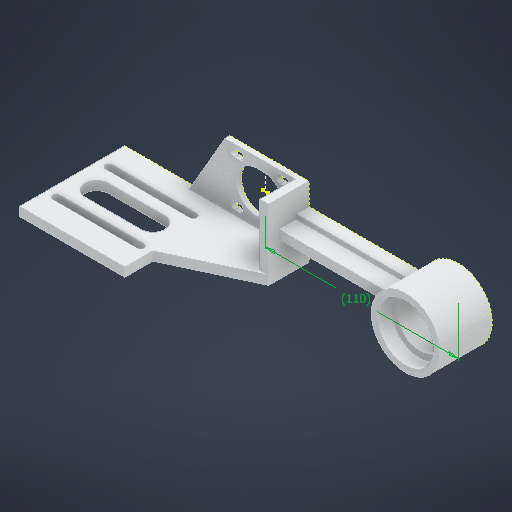
# Autodesk Inventor part: SupportV2_P2
Saved by Autodesk Inventor 2026.2 (Build 302298000, 298)
## iProperties
Created: 2023-04-27
Part Number: SupportV2_P2
Material: PET Plastic
Document SubType Name: Modeling
Designer: Vinicius Silva
Density: 1.541 g/cm^3
Appearance: White
Author: Vinicius Silva
Autodesk Inventor part; units mm, degrees
ref_plane "YZ Plane" through (0, 0, 0) normal (1, 0, 0) x (0, 1, 0)
ref_plane "XZ Plane" through (0, 0, 0) normal (0, 1, 0) x (-1, 0, 0)
ref_plane "XY Plane" through (0, 0, 0) normal (0, 0, 1) x (1, 0, 0)
sketch "Sketch1" plane through (0, 0, 0) normal (0, 0, 1) x (1, 0, 0)
  line L0 (0, 0) -> (30, 0)
  line L1 (30, 0) -> (30, 60)
  line L2 (30, 60) -> (0, 60)
  line L3 (6, 45) -> (24, 45) construction
  line L4 (6, 43) -> (24, 43)
  line L5 (24, 47) -> (6, 47)
  arc A0 (24, 43) -> (24, 47) centre (24, 45) ccw
  line L6 (6, 15) -> (24, 15) construction
  line L7 (6, 13) -> (24, 13)
  line L8 (24, 17) -> (6, 17)
  arc A1 (24, 13) -> (24, 17) centre (24, 15) ccw
  line L9 (0, 30) -> (16, 30) construction
  arc A2 (16, 23.25) -> (16, 36.75) centre (16, 30) ccw
  line L10 (0, 0) -> (-30, 0)
  line L11 (-30, 0) -> (-30, 60)
  line L12 (-30, 60) -> (0, 60)
  line L13 (-6, 45) -> (-24, 45) construction
  line L14 (24, 43) -> (-24, 43)
  line L15 (-24, 47) -> (24, 47)
  arc A3 (-24, 47) -> (-24, 43) centre (-24, 45) ccw
  line L16 (-6, 15) -> (-24, 15) construction
  line L17 (24, 13) -> (-24, 13)
  line L18 (-24, 17) -> (24, 17)
  arc A4 (-24, 17) -> (-24, 13) centre (-24, 15) ccw
  line L19 (0, 30) -> (-16, 30) construction
  arc A5 (-16, 36.75) -> (-16, 23.25) centre (-16, 30) ccw
  line L20 (-16, 36.75) -> (16, 36.75)
  line L21 (16, 23.25) -> (-16, 23.25)
  point P0 (15, 45)
  point P1 (15, 15)
  point P2 (8, 30)
  point P3 (-15, 50)
  point P4 (-15, 10)
  point P5 (-8, 30)
  dimension "d0" = 30
  dimension "d1" = 60
  dimension "d2" = 4
  dimension "d3" = 15
  dimension "d5" = 6
  dimension "d6" = 4
  dimension "d8" = 6
  dimension "d151" = 60
  dimension "d154" = 2
  dimension "d155" = 2
  dimension "d162" = 6
  dimension "d163" = 4
  dimension "d165" = 30
  dimension "d166" = 30
  dimension "d167" = 6
  dimension "d170" = 15
  dimension "d173" = 24
  dimension "d176" = 15
  dimension "d178" = 13.5
  dimension "d179" = 30
  constraints: 56 end point, 13 point on circle, 6 centre point, 5 parallel, 4 horizontal, 4 tangent, 3 midpoint, 2 collinear, 1 perpendicular
  measures "d0" distance of L2.end L1.end
  measures "d1" distance of L1.end L0.end
  measures "d2" diameter of A0
  measures "d3" distance between parallel lines of L2 L3
  measures "d5" distance from line of L1 L3.end
  measures "d6" diameter of A1
  measures "d8" distance from line of L1 L6.end
  measures "d151" distance between parallel lines of L1 L11
  measures "d154" radius of A4
  measures "d155" radius of A1
  measures "d162" distance from line of L13.end L11
  measures "d163" distance between parallel lines of L15 L14
  measures "d165" distance from line of L0.start L1
  measures "d166" distance from line of L11 L0.start
  measures "d167" distance from line of L11 L16.end
  measures "d170" distance from line of L12 L13.end
  measures "d173" horizontal distance of L0.start L13.end
  measures "d176" distance from line of L0 L6.end
  measures "d178" distance between parallel lines of L20 L21
  measures "d179" distance between parallel lines of L10 L19
extrude "Extrusion1" add sketch "Sketch1" along normal blind 5 contours L10 L11 L12 L2 L1 L0 | L21 A5 L20 A2
sketch "Sketch2" plane through (30, 0, 0) normal (1, 0, 0) x (0, 0, -1)
  line L0 (0, 60) -> (-5, 60) projected
  line L1 (0, 0) -> (0, 60) projected
  line L2 (0, 57) -> (-40, 57)
  line L3 (-40, 57) -> (-40, 60)
  line L4 (-40, 60) -> (0, 60)
  line L5 (0, 60) -> (0, 57)
  dimension "d12" = 40
  dimension "d13" = 3
  dimension "d16" = 0
  constraints: 8 end point, 2 parallel, 1 horizontal, 1 perpendicular, 1 point on line
  measures "d12" distance of L3.end L4.end
  measures "d13" distance of L2.end L3.end
  measures "d16" distance between parallel lines of L0 L4
extrude "Extrusion2" add sketch "Sketch2" along normal blind 45
draft "FaceDraft1" angle 30 pull direction (0, 0, 1) faces at (30, 58, 28.3333) fixed edges at (30, 58.5, 40)
sketch "Sketch4" plane through (75, 57, 5) normal (0, -1, 0) x (1, 0, 0)
  line L0 (0, 35) -> (-5, 35)
  line L1 (-5, 35) -> (-5, -5)
  line L2 (-5, -5) -> (0, -5)
  line L3 (0, -5) -> (0, 35)
  line L4 (-45, 35) -> (0, 35) construction
  line L5 (-105, -5) -> (0, -5) construction
  line L6 (-105, -5) -> (0, -5) construction
  line L7 (-65.2073, 0) -> (-105, 0) construction
  line L8 (-45, 35) -> (-65.2073, 0) construction
  line L9 (-45, 35) -> (0, 35) construction
  line L10 (0, -5) -> (0, 35) construction
  line L11 (-105, -5) -> (-105, 0) projected
  point P0 (-75, -5)
  point P1 (-5, 0)
  dimension "d136" = 40
  dimension "d137" = 5
  constraints: 8 end point, 2 parallel, 1 horizontal, 1 perpendicular
  measures "d136" distance between parallel lines of L4 L2
  measures "d137" distance between parallel lines of L1 L3
extrude "Extrusion4" add sketch "Sketch4" along normal blind 20
sketch "Sketch7" plane through (30, 60, 5) normal (0, 1, 0) x (1, 0, 0)
  line L0 (0, -35) -> (40, -35) construction
  line L1 (-20.2073, 0) -> (0, -35) construction
  line L2 (-20.2073, 0) -> (0, 0) construction
  line L3 (0, -35) -> (0, 0) construction
  line L4 (5.3, -30.6) -> (8.7, -30.6) construction
  line L5 (5.3, -32.8) -> (8.7, -32.8)
  line L6 (8.7, -28.4) -> (5.3, -28.4)
  arc A0 (5.3, -28.4) -> (5.3, -32.8) centre (5.3, -30.6) ccw
  arc A1 (8.7, -32.8) -> (8.7, -28.4) centre (8.7, -30.6) ccw
  line L7 (5.3, -4.6) -> (8.7, -4.6) construction
  line L8 (5.3, -6.8) -> (8.7, -6.8)
  line L9 (8.7, -2.4) -> (5.3, -2.4)
  arc A2 (5.3, -2.4) -> (5.3, -6.8) centre (5.3, -4.6) ccw
  arc A3 (8.7, -6.8) -> (8.7, -2.4) centre (8.7, -4.6) ccw
  line L10 (31.3, -30.6) -> (34.7, -30.6) construction
  line L11 (31.3, -32.8) -> (34.7, -32.8)
  line L12 (34.7, -28.4) -> (31.3, -28.4)
  arc A4 (31.3, -28.4) -> (31.3, -32.8) centre (31.3, -30.6) ccw
  arc A5 (34.7, -32.8) -> (34.7, -28.4) centre (34.7, -30.6) ccw
  line L13 (31.3, -4.6) -> (34.7, -4.6) construction
  line L14 (31.3, -6.8) -> (34.7, -6.8)
  line L15 (34.7, -2.4) -> (31.3, -2.4)
  arc A6 (31.3, -2.4) -> (31.3, -6.8) centre (31.3, -4.6) ccw
  arc A7 (34.7, -6.8) -> (34.7, -2.4) centre (34.7, -4.6) ccw
  line L16 (18.5, -17.5) -> (21.5, -17.5) construction
  line L17 (18.5, -29.5) -> (21.5, -29.5)
  line L18 (21.5, -5.5) -> (18.5, -5.5)
  arc A8 (18.5, -5.5) -> (18.5, -29.5) centre (18.5, -17.5) ccw
  arc A9 (21.5, -29.5) -> (21.5, -5.5) centre (21.5, -17.5) ccw
  line L19 (18.5, -17.5) -> (21.5, -17.5) construction
  line L20 (0, -17.5) -> (40, -17.5) construction
  line L21 (20, -35) -> (20, 0) construction
  line L22 (0, 5) -> (0, 0) projected
  line L23 (0, 5) -> (40, 5) projected
  line L24 (40, 5) -> (40, -35) projected
  line L25 (-30, 5) -> (45, 5) construction
  line L26 (45, 5) -> (45, -35) construction
  line L27 (40, -35) -> (40, 5) construction
  line L28 (0, -35) -> (45, -35) construction
  line L29 (-30, 5) -> (0, 5) construction
  line L30 (0, 5) -> (0, -35) construction
  line L31 (-20.2073, 0) -> (0, -35) construction
  line L32 (0, -35) -> (45, -35) construction
  line L33 (45, -35) -> (45, 5) construction
  line L34 (45, 5) -> (0, 5) construction
  point P0 (7, -30.6)
  point P1 (7, -4.6)
  point P2 (33, -30.6)
  point P3 (33, -4.6)
  point P4 (20, -17.5)
  point P5 (20, -17.5)
  dimension "d37" = 26
  dimension "d40" = 26
  dimension "d45" = 24
  dimension "d138" = 4.4
  dimension "d139" = 7
  dimension "d140" = 3.4
  dimension "d141" = 3
  dimension "d142" = 5.5
  dimension "d143" = 6.6
  dimension "d144" = 20
  constraints: 56 end point, 20 point on circle, 10 centre point, 8 tangent, 5 horizontal, 5 midpoint, 3 perpendicular, 2 collinear, 2 parallel, 1 vertical, 36 other
  measures "d37" distance of L5.start L8.start
  measures "d40" distance of L5.start L11.start
  measures "d45" diameter of A9
  measures "d138" distance from line of L0 point (7, -30.6)
  measures "d139" distance from line of L3 point (7, -30.6)
  measures "d140" distance of L5.start L5.end
  measures "d141" distance of L17.start L17.end
  measures "d142" distance between parallel lines of L0 L17
  measures "d143" distance between parallel lines of L0 L6
  measures "d144" distance from line of L3 point (20, -17.5)
extrude "Extrusion5" cut sketch "Sketch7" against normal blind 5
sketch "Sketch13" plane through (75, 0, 0) normal (1, 0, 0) x (0, 0, -1)
  line L0 (-40, 57) -> (-40, 60) construction
  line L1 (-40, 60) -> (-5, 60) construction
  line L2 (-34.5, 60) -> (-10.5, 60) construction
  line L3 (-17.5, 52.5) -> (-17.5, 60)
  line L4 (-17.5, 60) -> (-27.5, 60)
  line L5 (-27.5, 60) -> (-27.5, 52.5)
  line L6 (-20, 52.5) -> (-20, 42.5)
  line L7 (-20, 42.5) -> (-25, 42.5)
  line L8 (-25, 42.5) -> (-25, 52.5)
  line L9 (-27.5, 52.5) -> (-25, 52.5)
  line L10 (-20, 52.5) -> (-17.5, 52.5)
  line L11 (0, 60) -> (0, 37) construction
  line L12 (0, 60) -> (-40, 60) construction
  line L13 (-40, 60) -> (-40, 37) construction
  line L14 (0, 37) -> (-40, 37) construction
  line L15 (-34.5, 60) -> (-10.5, 60) construction
  line L16 (-22.5, 60) -> (-22.5, 37) construction
  point P0 (0, 0)
  point P1 (-5, 9)
  dimension "d69" = 5
  dimension "d126" = 7.5
  dimension "d127" = 7.5
  dimension "d128" = 10
  dimension "d132" = 5
  dimension "d133" = 5
  dimension "d134" = 2.5
  dimension "d135" = 2.5
  constraints: 20 end point, 4 parallel, 3 horizontal, 3 perpendicular, 2 point on line, 1 midpoint
  measures "d69" distance of L6.end L7.end
  measures "d126" distance of L3.start L3.end
  measures "d127" distance of L4.end L5.end
  measures "d128" distance of L6.start L6.end
  measures "d132" distance from line of L3 L16.start
  measures "d133" distance between parallel lines of L16 L5
  measures "d134" distance between parallel lines of L16 L8
  measures "d135" distance between parallel lines of L16 L6
extrude "Extrusion23" add sketch "Sketch13" along normal blind 66.152
sketch "Sketch31" plane through (30, 60, 5) normal (0, 1, 0) x (0.8660254, 0, -0.5)
  line L0 (86.2605, -72.8965) -> (88.7605, -68.5664) construction
  line L1 (88.7605, -68.5664) -> (90.0105, -66.4013) construction
  line L2 (85.0105, -75.0616) -> (86.2605, -72.8965) construction
  circle A0 centre (103.8334, -80.1555) radius 19.5
  circle A1 centre (103.8334, -80.1555) radius 16
  point P0 (-23.4808, 19.3301)
  dimension "d114" = 39
  dimension "d115" = 32
  constraints: 2 centre point, 2 point on circle, 1 coincident
  measures "d114" diameter of A0
  measures "d115" diameter of A1
extrude "Extrusion24" add sketch "Sketch31" against normal blind 30
sketch "Sketch34" plane through (0, 0, 0) normal (0, 0, -1) x (-1, 0, 0)
  arc A0 (-24, 17) -> (-24, 13) centre (-24, 15) ccw construction
  arc A1 (-24, 47) -> (-24, 43) centre (-24, 45) ccw construction
  line L0 (30, 0) -> (-30, 0) construction
  line L1 (30, 60) -> (-75, 60) construction
  line L2 (-75, 60) -> (-75, 37) construction
  line L3 (-70, 37) -> (-75, 37) construction
  line L4 (-70, 57) -> (-70, 37) construction
  line L5 (-30, 57) -> (-70, 57) construction
  line L6 (-30, 0) -> (-30, 57) construction
  line L7 (-75, 37) -> (-30, 16.0162)
  line L8 (-75, 37) -> (-25.348, 37) construction
  line L9 (-75, 60) -> (-75, 37) projected
  line L10 (-75, 37) -> (-75, 57)
  line L11 (-30, 57) -> (-70, 57) projected
  line L12 (-75, 57) -> (-30, 57)
  line L13 (-30, 57) -> (-30, 16.0162)
  line L14 (-24, 17) -> (24, 17) projected
  arc A2 (24, 13) -> (24, 17) centre (24, 15) ccw projected
  line L15 (24, 13) -> (-24, 13) projected
  arc A3 (24, 43) -> (24, 47) centre (24, 45) ccw projected
  line L16 (24, 43) -> (-24, 43) projected
  line L17 (-24, 47) -> (24, 47) projected
  line L18 (30, 60) -> (30, 0) projected
  point P0 (0, 0)
  dimension "d129" = 25
  constraints: 10 end point, 2 horizontal, 2 point on line, 1 equal length, 1 perpendicular
  measures "d129" angle of L7 L8
extrude "Extrusion26" add sketch "Sketch34" against normal blind 5
ref_plane "Work Plane9" through (160.0001, 50, 22.5) normal (0, 1, 0) x (1, 0, 0)
extrude "Extrusion28" cut sketch "Sketch1" along normal blind 10 contours L21 A5 L20 A2
sketch "Sketch36" plane through (-30, 60, 5) normal (0, 1, 0) x (1, 0, 0)
  arc A0 (171.152, -22.5) -> (171.152, -12.5) centre (190.0001, -17.5) ccw construction
  line L0 (105, -12.5) -> (171.152, -12.5) construction
  line L1 (105, 5) -> (105, -12.5) construction
  line L2 (0, 5) -> (105, 5) construction
  line L3 (0, 5) -> (0, 0) construction
  line L4 (39.7927, 0) -> (0, 0) construction
  line L5 (60, -35) -> (39.7927, 0) construction
  line L6 (60, -35) -> (105, -35) construction
  line L7 (105, -22.5) -> (105, -35) construction
  line L8 (105, -22.5) -> (171.152, -22.5) construction
  arc A1 (81.5, -29.5) -> (81.5, -5.5) centre (81.5, -17.5) ccw construction
  line L9 (81.5, -29.5) -> (78.5, -29.5) construction
  arc A2 (78.5, -5.5) -> (78.5, -29.5) centre (78.5, -17.5) ccw construction
  line L10 (78.5, -5.5) -> (81.5, -5.5) construction
  arc A3 (94.7, -32.8) -> (94.7, -28.4) centre (94.7, -30.6) ccw construction
  line L11 (94.7, -32.8) -> (91.3, -32.8) construction
  arc A4 (91.3, -28.4) -> (91.3, -32.8) centre (91.3, -30.6) ccw construction
  line L12 (91.3, -28.4) -> (94.7, -28.4) construction
  arc A5 (68.7, -32.8) -> (68.7, -28.4) centre (68.7, -30.6) ccw construction
  line L13 (68.7, -32.8) -> (65.3, -32.8) construction
  arc A6 (65.3, -28.4) -> (65.3, -32.8) centre (65.3, -30.6) ccw construction
  line L14 (65.3, -28.4) -> (68.7, -28.4) construction
  arc A7 (68.7, -6.8) -> (68.7, -2.4) centre (68.7, -4.6) ccw construction
  line L15 (68.7, -6.8) -> (65.3, -6.8) construction
  arc A8 (65.3, -2.4) -> (65.3, -6.8) centre (65.3, -4.6) ccw construction
  line L16 (65.3, -2.4) -> (68.7, -2.4) construction
  arc A9 (94.7, -6.8) -> (94.7, -2.4) centre (94.7, -4.6) ccw construction
  line L17 (94.7, -6.8) -> (91.3, -6.8) construction
  arc A10 (91.3, -2.4) -> (91.3, -6.8) centre (91.3, -4.6) ccw construction
  line L18 (91.3, -2.4) -> (94.7, -2.4) construction
  line L19 (80, -5.5) -> (80, -29.5) construction
  point P0 (30, 5)
  dimension "d177" = 110.0001
  constraints: 2 end point, 2 midpoint
  measures "d177" distance from line of A0.centre L19
ref_plane "Work Plane10" through (-30, 45, 0) normal (0, 1, 0) x (1, 0, 0)
sketch "Sketch37" plane through (-30, 45, 0) normal (0, 1, 0) x (1, 0, 0)
  circle A0 centre (190.0001, -22.5) radius 16 projected
  circle A1 centre (190.0001, -22.5) radius 13
  point P0 (30, 0)
  dimension "d180" = 3
  constraints: 1 centre point
  measures "d180" radial gap between concentric circles of A0 A1
extrude "Extrusion29" add sketch "Sketch37" along normal mid plane 14
body "Solid1"
